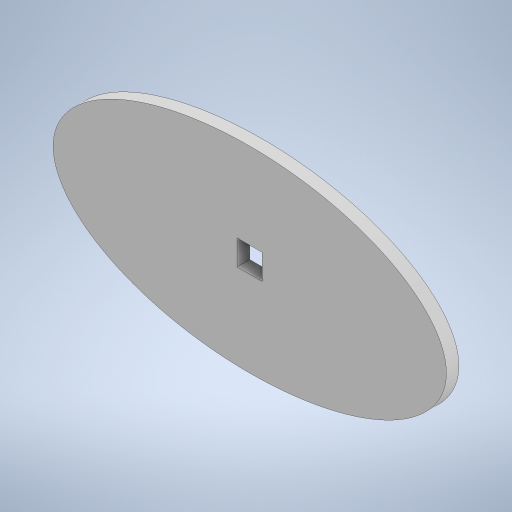
# Autodesk Inventor part: arms front
Saved by Autodesk Inventor 2023 (Build 270158000, 158)
## iProperties
Created: 2023-11-14
Part Number: arms front
Material: Generic
Document SubType Name: Modeling
Designer: Nate
Density: 1 g/cm^3
Appearance: Default
Author: Nate
Autodesk Inventor part; units mm, degrees
ref_plane "YZ Plane" through (0, 0, 0) normal (1, 0, 0) x (0, 1, 0)
ref_plane "XZ Plane" through (0, 0, 0) normal (0, 1, 0) x (-1, 0, 0)
ref_plane "XY Plane" through (0, 0, 0) normal (0, 0, 1) x (1, 0, 0)
sketch "Sketch1" plane through (0, 0, 0) normal (0, 0, 1) x (1, 0, 0)
  ellipse E0 centre (0, 0) end of major axis (0, -25) minor radius 50
  line L0 (-3.175, 3.175) -> (3.175, 3.175)
  line L1 (3.175, 3.175) -> (3.175, -3.175)
  line L2 (3.175, -3.175) -> (-3.175, -3.175)
  line L3 (-3.175, -3.175) -> (-3.175, 3.175)
  line L4 (-3.175, 3.175) -> (3.175, -3.175) construction
  line L5 (3.175, 3.175) -> (-3.175, -3.175) construction
  dimension "d1" = 25
  dimension "d2" = 50
  dimension "d3" = 6.35
  dimension "d4" = 6.35
  constraints: 12 end point, 2 midpoint, 2 parallel, 1 coincident, 1 horizontal, 1 perpendicular, 2 other
  measures "d3" distance between parallel lines of L1 L3
  measures "d4" distance between parallel lines of L2 L0
extrude "Extrusion1" add sketch "Sketch1" along normal blind 3.175
body "Solid1"
